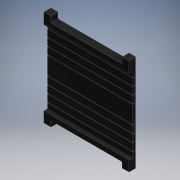
# Autodesk Inventor part: -Y
Saved by Autodesk Inventor 2018 (Build 220112000, 112)
## iProperties
Created: 2018-07-04
Part Number: -Y
Material: Aluminum 6061
Document SubType Name: Modeling
Designer: Bradley
Density: 2.7 g/cm^3
Appearance: Anodized - Dark Gray
Author: Bradley
Autodesk Inventor part; units mm, degrees
ref_plane "YZ Plane" through (0, 0, 0) normal (1, 0, 0) x (0, 1, 0)
ref_plane "XZ Plane" through (0, 0, 0) normal (0, 1, 0) x (-1, 0, 0)
ref_plane "XY Plane" through (0, 0, 0) normal (0, 0, 1) x (1, 0, 0)
sketch "Sketch1" plane through (0, 0, 0) normal (0, 1, 0) x (-1, 0, 0)
  line L0 (50, 57) -> (50, -56.5)
  line L1 (50, -56.5) -> (41.5, -56.5)
  line L2 (41.5, -56.5) -> (41.5, -50)
  line L3 (41.5, -50) -> (-41.5, -50)
  line L4 (-41.5, -50) -> (-41.5, -56.5)
  line L5 (-41.5, -56.5) -> (-50, -56.5)
  line L6 (-50, -56.5) -> (-50, 57)
  line L7 (-50, 57) -> (-41.5, 57)
  line L8 (-41.5, 57) -> (-41.5, 50)
  line L9 (-41.5, 50) -> (41.5, 50)
  line L10 (41.5, 50) -> (41.5, 57)
  line L11 (50, 57) -> (41.5, 57)
  point P0 (0, 0)
  point P1 (0, 0)
  point P2 (0, 50)
  dimension "d0" = 100
  dimension "d1" = 8.5
  dimension "d2" = 113.5
  dimension "d3" = 7
  dimension "d4" = 6.5
  dimension "d5" = 56.5
  constraints: 24 end point, 8 perpendicular, 7 point on line, 1 coincident, 1 collinear, 1 midpoint, 1 vertical, 1 vertical alignment
  measures "d0" distance between parallel lines of L6 L0
  measures "d1" distance of L0.start L10.end
  measures "d2" distance of L0.start L0.end
  measures "d3" distance of L9.end L10.end
  measures "d4" distance of L1.end L2.end
  measures "d5" distance from line of point (0, 0) L1
extrude "Extrusion1" add sketch "Sketch1" along normal mid plane 8.5
sketch "Sketch2" plane through (50, -4.25, -56.5) normal (1, 0, 0) x (0, 0, -1)
  line L0 (0, 8.5) -> (0, 0) projected
  line L1 (-113.5, 8.5) -> (0, 8.5) projected
  line L2 (-113.5, 8.5) -> (-113.5, 0) projected
  line L3 (0, 0) -> (-113.5, 0) projected
  line L4 (-106.5, 8.5) -> (-106.5, 0) projected
  line L5 (-6.5, 8.5) -> (-6.5, 0) projected
  line L6 (0, 0) -> (-113.5, 0) projected
  line L7 (-100.5, 0) -> (-100.5, 4.5)
  line L8 (-100.5, 4.5) -> (-12.5, 4.5)
  line L9 (-12.5, 4.5) -> (-12.5, 0)
  line L10 (-46.6, 4.5) -> (-45.4, 4.5)
  line L11 (-45.4, 4.5) -> (-45.4, 6.5)
  line L12 (-45.4, 6.5) -> (-46.6, 6.5)
  line L13 (-46.6, 6.5) -> (-46.6, 4.5)
  line L14 (0, 8.5) -> (-113.5, 8.5) construction
  line L15 (-56.5, 8.5) -> (-56.5, 0) construction
  line L16 (-36.4, 4.5) -> (-36.4, 6.5)
  line L17 (-37.6, 4.5) -> (-36.4, 4.5)
  line L18 (-37.6, 6.5) -> (-37.6, 4.5)
  line L19 (-36.4, 6.5) -> (-37.6, 6.5)
  line L20 (-27.4, 4.5) -> (-27.4, 6.5)
  line L21 (-28.6, 4.5) -> (-27.4, 4.5)
  line L22 (-28.6, 6.5) -> (-28.6, 4.5)
  line L23 (-27.4, 6.5) -> (-28.6, 6.5)
  line L24 (-18.4, 4.5) -> (-18.4, 6.5)
  line L25 (-19.6, 4.5) -> (-18.4, 4.5)
  line L26 (-19.6, 6.5) -> (-19.6, 4.5)
  line L27 (-18.4, 6.5) -> (-19.6, 6.5)
  line L28 (-66.4, 4.5) -> (-67.6, 4.5)
  line L29 (-67.6, 4.5) -> (-67.6, 6.5)
  line L30 (-67.6, 6.5) -> (-66.4, 6.5)
  line L31 (-66.4, 6.5) -> (-66.4, 4.5)
  line L32 (-76.6, 4.5) -> (-76.6, 6.5)
  line L33 (-75.4, 4.5) -> (-76.6, 4.5)
  line L34 (-75.4, 6.5) -> (-75.4, 4.5)
  line L35 (-76.6, 6.5) -> (-75.4, 6.5)
  line L36 (-85.6, 4.5) -> (-85.6, 6.5)
  line L37 (-84.4, 4.5) -> (-85.6, 4.5)
  line L38 (-84.4, 6.5) -> (-84.4, 4.5)
  line L39 (-85.6, 6.5) -> (-84.4, 6.5)
  line L40 (-94.6, 4.5) -> (-94.6, 6.5)
  line L41 (-93.4, 4.5) -> (-94.6, 4.5)
  line L42 (-93.4, 6.5) -> (-93.4, 4.5)
  line L43 (-94.6, 6.5) -> (-93.4, 6.5)
  point P0 (-56.5, 4.25)
  point P1 (-56.5, 4.25)
  point P2 (-46, 6.5)
  point P3 (-37, 6.5)
  point P4 (-28, 6.5)
  point P5 (-19, 6.5)
  point P6 (-67, 6.5)
  point P7 (-76, 6.5)
  point P8 (-85, 6.5)
  point P9 (-94, 6.5)
  dimension "d8" = 4
  dimension "d9" = 6
  dimension "d10" = 6
  dimension "d11" = 1.2
  dimension "d14" = 9
  dimension "d19" = 21
  dimension "d20" = 2
  constraints: 72 end point, 20 symmetric about line, 5 point on line, 4 perpendicular, 3 parallel, 2 horizontal, 2 midpoint, 1 coincident, 27 other
  measures "d8" distance between parallel lines of L1 L8
  measures "d9" distance between parallel lines of L7 L4
  measures "d10" distance between parallel lines of L5 L9
  measures "d11" distance of L11.end L12.end
  measures "d14" distance of L11.end L16.end
  measures "d19" distance of point (-46, 6.5) point (-67, 6.5)
  measures "d20" distance between parallel lines of L1 L12
extrude "Extrusion2" cut sketch "Sketch2" against normal through all contours L3 L7 L8 L9 | L8 L26 L27 L24 | L40 L43 L42 L8 | L8 L22 L23 L20 | L36 L39 L38 L8 | L8 L18 L19 L16 | L32 L35 L34 L8 | L8 L13 L12 L11 | L29 L30 L31 L8
fillet "Fillet1" radius 1 6 edges at (41.5, 0, 50) (-41.5, 0, 50) (-41.5, 0, -50) (41.5, 0, -50) (50, 4.25, 0.25) (-50, 4.25, 0.25)
chamfer "Chamfer1" distance 0.5 angle 45 40 edges at (45.75, -4.25, 57) (41.5, 0, 57) (49.7071, 3.9571, 57) (50, -0.5, 57) (45.25, 4.25, 57) (-45.25, 4.25, 57) (-49.7071, 3.9571, 57) (-50, -0.5, 57) (-41.5, 0, 57) (-45.75, -4.25, 57) (-41.5, 0, -56.5) (-45.75, -4.25, -56.5) (-45.25, 4.25, -56.5) (-49.7071, 3.9571, -56.5) (-50, -0.5, -56.5) (50, -0.5, -56.5) (49.7071, 3.9571, -56.5) (45.25, 4.25, -56.5) (41.5, 0, -56.5) (45.75, -4.25, -56.5) (0, 4.25, -50) (-41.2071, 4.25, -50.2929) (-41.5, 4.25, -53.75) (41.2071, 4.25, -50.2929) (41.5, 4.25, -53.75) (0, 4.25, 50) (41.2071, 4.25, 50.2929) (41.5, 4.25, 54) (-41.2071, 4.25, 50.2929) (-41.5, 4.25, 54) (0, -4.25, 50) (-41.2071, -4.25, 50.2929) (-41.5, -4.25, 54) (41.2071, -4.25, 50.2929) (41.5, -4.25, 54) (-41.2071, -4.25, -50.2929) (-41.5, -4.25, -53.75) (0, -4.25, -50) (41.2071, -4.25, -50.2929) (41.5, -4.25, -53.75)
body "Solid1"
